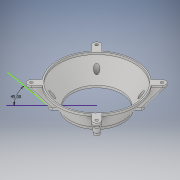
# Autodesk Inventor part: vents - 7-27
Saved by Autodesk Inventor 2018.1 (Build 221156000, 156)
## iProperties
Created: 2017-06-19
Part Number: vents - 7-27
Material: Generic
Document SubType Name: Modeling
Designer: admin1
Density: 1 g/cm^3
Appearance: Default
Author: admin1
Autodesk Inventor part; units mm, degrees
ref_plane "YZ Plane" through (0, 0, 0) normal (1, 0, 0) x (0, 1, 0)
ref_plane "XZ Plane" through (0, 0, 0) normal (0, 1, 0) x (-1, 0, 0)
ref_plane "XY Plane" through (0, 0, 0) normal (0, 0, 1) x (1, 0, 0)
sketch "Cowling_sketch" plane through (0, 0, 0) normal (0, 1, 0) x (-1, 0, 0)
  line L0 (11.6642, 0) -> (-13.8582, 0) construction
  line L1 (0, -40) -> (28.563, -60)
  line L2 (28.563, -60) -> (28.563, -62)
  line L3 (28.563, -62) -> (0, -42)
  line L4 (0, -42) -> (0, -40)
  line L5 (0, 0) -> (0, -166.056) construction
  line L6 (61.4713, 0) -> (-26.4131, 0) projected
  dimension "smallsize" = 40
  dimension "largesize" = 60
  dimension "cowlingangle" = 55
  dimension "wallthickness" = 2
  constraints: 12 end point, 2 horizontal, 2 parallel, 2 vertical, 1 point on line
  measures "smallsize" distance from line of L0 L1.start
  measures "largesize" distance from line of L0 L1.end
  measures "cowlingangle" angle of L3 L5
  measures "wallthickness" distance of L3.end L1.start
revolve "Cowling_revolution" add sketch "Cowling_sketch" angle 360 about axis through (-10, 0, 0) along (1, 0, 0)
sketch "LargeFlange_sketch" plane through (-28.563, 0, 0) normal (-1, 0, 0) x (0, 0, 1)
  circle A0 centre (0, 0) radius 60
  circle A1 centre (0, 0) radius 60 projected
  circle A2 centre (0, 0) radius 62 projected
  line L0 (0, 0) -> (0, -145.4431) construction
  line L1 (0, 0) -> (117.2318, 0) construction
  line L2 (0, 0) -> (87.9805, -87.9805) construction
  arc A3 (48.4341, -56.5659) -> (56.5659, -48.4341) centre (52.5, -52.5) ccw
  line L3 (48.4341, -56.5659) -> (39.5858, -47.7175)
  line L4 (56.5659, -48.4341) -> (47.7175, -39.5858)
  arc A4 (56.5659, 48.4341) -> (48.4341, 56.5659) centre (52.5, 52.5) ccw
  line L5 (48.4341, 56.5659) -> (39.5858, 47.7175)
  line L6 (56.5659, 48.4341) -> (47.7175, 39.5858)
  arc A5 (-48.4341, 56.5659) -> (-56.5659, 48.4341) centre (-52.5, 52.5) ccw
  line L7 (-56.5659, 48.4341) -> (-47.7175, 39.5858)
  line L8 (-48.4341, 56.5659) -> (-39.5858, 47.7175)
  arc A6 (-56.5659, -48.4341) -> (-48.4341, -56.5659) centre (-52.5, -52.5) ccw
  line L9 (-48.4341, -56.5659) -> (-39.5858, -47.7175)
  line L10 (-56.5659, -48.4341) -> (-47.7175, -39.5858)
  arc A7 (-39.5858, -47.7175) -> (39.5858, -47.7175) centre (0, 0) ccw
  arc A8 (-47.7175, 39.5858) -> (-47.7175, -39.5858) centre (0, 0) ccw
  arc A9 (47.7175, -39.5858) -> (47.7175, 39.5858) centre (0, 0) ccw
  arc A10 (39.5858, 47.7175) -> (-39.5858, 47.7175) centre (0, 0) ccw
  dimension "d8" = 45
  dimension "d9" = 11.5
  dimension "d12" = 360
  dimension "largeholes" = 52.5
  dimension "d15" = 52.5
  constraints: 22 end point, 18 point on circle, 9 centre point, 2 coincident, 2 concentric, 2 horizontal, 2 parallel, 2 point on line, 2 tangent, 2 vertical, 33 other
  measures "d8" angle of L0 L2
  measures "d9" diameter of A3
  measures "largeholes" distance from line of L0 A3.centre
  measures "d15" distance from line of L1 A3.centre
extrude "LargeFlange_extrude" add sketch "LargeFlange_sketch" along normal blind 3.5
sketch "SmallFlange_sketch" plane through (0, 0, 0) normal (1, 0, 0) x (0, 0, -1)
  circle A0 centre (0, 0) radius 40
  circle A1 centre (0, 0) radius 40 projected
  circle A2 centre (0, 0) radius 42 projected
  line L0 (0, 0) -> (0, 99.3932) construction
  line L1 (0, 0) -> (-104.4919, 0) construction
  line L2 (0, 0) -> (-82.1484, 82.1484) construction
  arc A3 (-32.8332, 38.6668) -> (-38.6668, 32.8332) centre (-35.75, 35.75) ccw
  line L3 (-32.8332, 38.6668) -> (-26.6381, 32.4717)
  line L4 (-38.6668, 32.8332) -> (-32.4717, 26.6381)
  arc A4 (-38.6668, -32.8332) -> (-32.8332, -38.6668) centre (-35.75, -35.75) ccw
  line L5 (-38.6668, -32.8332) -> (-32.4717, -26.6381)
  line L6 (-32.8332, -38.6668) -> (-26.6381, -32.4717)
  arc A5 (32.8332, -38.6668) -> (38.6668, -32.8332) centre (35.75, -35.75) ccw
  line L7 (32.8332, -38.6668) -> (26.6381, -32.4717)
  line L8 (38.6668, -32.8332) -> (32.4717, -26.6381)
  arc A6 (38.6668, 32.8332) -> (32.8332, 38.6668) centre (35.75, 35.75) ccw
  line L9 (38.6668, 32.8332) -> (32.4717, 26.6381)
  line L10 (32.8332, 38.6668) -> (26.6381, 32.4717)
  arc A7 (26.6381, 32.4717) -> (-26.6381, 32.4717) centre (0, 0) ccw
  arc A8 (32.4717, -26.6381) -> (32.4717, 26.6381) centre (0, 0) ccw
  arc A9 (-32.4717, 26.6381) -> (-32.4717, -26.6381) centre (0, 0) ccw
  arc A10 (-26.6381, -32.4717) -> (26.6381, -32.4717) centre (0, 0) ccw
  dimension "d18" = 45
  dimension "smallholes" = 35.75
  dimension "d20" = 8.25
  dimension "d23" = 360
  constraints: 22 end point, 18 point on circle, 9 centre point, 3 point on line, 2 coincident, 2 concentric, 2 horizontal, 2 parallel, 2 tangent, 2 vertical, 33 other
  measures "d18" angle of L0 L2
  measures "smallholes" distance from line of L0 A3.centre
  measures "d20" diameter of A3
extrude "SmallFlange_extrude" add sketch "SmallFlange_sketch" along normal blind 3.5
sketch "CowlingSlope_UpperPattern_sketch" plane through (-28.563, 0, 0) normal (1, 0, 0) x (0, 0, -1)
  arc A0 (-56.5659, -48.4341) -> (-48.4341, -56.5659) centre (-52.5, -52.5) ccw
  arc A1 (-56.5659, -48.4341) -> (-48.4341, -56.5659) centre (-52.5, -52.5) ccw projected
  line L0 (-56.5659, -48.4341) -> (-47.7175, -39.5858)
  arc A2 (-47.7175, -39.5858) -> (-39.5858, -47.7175) centre (0, 0) ccw projected
  line L1 (-56.5659, -48.4341) -> (-47.7175, -39.5858) projected
  line L2 (-48.4341, -56.5659) -> (-39.5858, -47.7175)
  line L3 (-39.5858, -47.7175) -> (-48.4341, -56.5659) projected
  line L4 (-47.7175, -39.5858) -> (-39.5858, -47.7175)
  point P0 (-55.0385, -28.5441)
  point P1 (-28.5441, -55.0385)
  point P2 (55.0385, 28.5441)
  point P3 (28.5441, 55.0385)
  constraints: 6 end point, 4 point on circle, 2 collinear, 2 tangent, 1 centre point, 1 point on line, 3 other
sketch "CowlingSlope_LowerPattern_sketch" plane through (0, 0, 0) normal (-1, 0, 0) x (0, 0, 1)
  arc A0 (32.8332, -38.6668) -> (38.6668, -32.8332) centre (35.75, -35.75) ccw
  arc A1 (32.8332, -38.6668) -> (38.6668, -32.8332) centre (35.75, -35.75) ccw projected
  line L0 (32.8332, -38.6668) -> (26.6381, -32.4717)
  arc A2 (26.6381, -32.4717) -> (32.4717, -26.6381) centre (0, 0) ccw projected
  line L1 (32.8332, -38.6668) -> (26.6381, -32.4717) projected
  line L2 (38.6668, -32.8332) -> (32.4717, -26.6381)
  line L3 (32.4717, -26.6381) -> (38.6668, -32.8332) projected
  line L4 (26.6381, -32.4717) -> (32.4717, -26.6381)
  constraints: 8 end point, 4 point on circle, 2 collinear, 2 concentric, 2 tangent, 1 centre point
loft "CowlingSlope_loft" add section 1 edges at (-28.563, -43.8406, 43.8406) (-28.563, -44.01, 52.1417) (-28.563, -56.5659, 56.5659) (-28.563, -52.1417, 44.01) section 2 edges at (0, -29.6985, 29.6985) (0, -35.5693, 29.7356) (0, -38.6668, 38.6668) (0, -29.7356, 35.5693)
hole "LargeScrewhole" at (-32.063, -52.5, 52.5) direction (1, 0, 0) diameter 4.5 depth 3.5
hole "LargeCounterbore" at (-28.563, -52.5, 52.5) direction (1, 0, 0) diameter 7.5 end through all
hole "SmallScrewhole" at (3.5, -35.75, 35.75) direction (-1, 0, 0) diameter 4.5 depth 3.5
hole "SmallCounterbore" at (0, -35.75, 35.75) direction (-1, 0, 0) diameter 7.5 end through all
pattern_circular "CowlingSlope_pattern" count 4 over 360 about axis through (-10, 0, 0) along (1, 0, 0) of "CowlingSlope_loft", "LargeScrewhole", "LargeCounterbore", "SmallScrewhole", "SmallCounterbore"
ref_plane "Work Plane3" through (-32.063, -56.5659, 56.5659) normal (0, -0.7071068, -0.7071068) x (0, 0.7071068, -0.7071068)
sketch "Sketch8" plane through (-32.063, -56.5659, 56.5659) normal (0, -0.7071068, -0.7071068) x (0, 0.7071068, -0.7071068)
  line L0 (79.9962, 32.063) -> (-22.7919, 32.063)
  line L1 (25.1096, 32.063) -> (-21.7168, -14.7635)
  dimension "d87" = 45
  constraints: 4 end point, 1 horizontal, 1 point on line
  measures "d87" angle of L0 L1
equation "\"d9\" = 2 * wallthickness + largesize - largeholes"
equation "\"d15\" = largeholes"
equation "\"d20\" = 2 * wallthickness + smallsize - smallholes"
equation "\"d47\" = largeflange"
equation "\"d67\" = smallflange"
equation "\"d76\" = smallflange"
equation "\"largeflange\" = 3.5"
equation "\"smallflange\" = 3.5"
body "Solid1"
